Autodesk Inventor part; units mm, degrees
(part 2 of 7)
sketch "Sketch1" plane through (0, 0, 0) normal (0, 0, 1) x (1, 0, 0)
  circle A0 centre (3.25, 6.65) radius 1.2295 projected
  line L0 (0, 0) -> (6.5, 0) projected
  line L1 (6.5, 0) -> (6.5, 9.3) projected
  line L2 (6.5, 9.3) -> (0, 9.3) projected
  line L3 (0, 0) -> (0, 9.3) projected
  circle A1 centre (3.25, 13.15) radius 1.2295 projected
  line L4 (0, 9.3) -> (6.5, 9.3) projected
  line L5 (6.5, 9.3) -> (6.5, 17) projected
  line L6 (0, 17) -> (6.5, 17) projected
  line L7 (0, 9.3) -> (0, 17) projected
  circle A2 centre (-9.75, 13.15) radius 1.2295 projected
  line L8 (-41.3371, 11.3) -> (-13, 11.3) projected
  line L9 (-41.3371, 9.3) -> (-41.3371, 11.3) projected
  line L10 (-41.3371, 9.3) -> (-6.5, 9.3) projected
  line L11 (-6.5, 9.3) -> (-6.5, 17) projected
  line L12 (-13, 17) -> (-6.5, 17) projected
  line L13 (-13, 11.3) -> (-13, 17) projected
  circle A3 centre (-9.75, -51.55) radius 1.2295 projected
  line L14 (-41.3371, -47.7) -> (-6.5, -47.7) projected
  line L15 (-41.3371, -47.7) -> (-41.3371, -49.7) projected
  line L16 (-13, -49.7) -> (-41.3371, -49.7) projected
  line L17 (-13, -49.7) -> (-13, -55.4) projected
  line L18 (-6.5, -55.4) -> (-13, -55.4) projected
  line L19 (-6.5, -47.7) -> (-6.5, -55.4) projected
  circle A4 centre (3.25, -51.55) radius 1.2295 projected
  line L20 (0, -47.7) -> (6.5, -47.7) projected
  line L21 (0, -47.7) -> (0, -55.4) projected
  line L22 (6.5, -55.4) -> (0, -55.4) projected
  line L23 (6.5, -47.7) -> (6.5, -55.4) projected
  circle A5 centre (3.25, -45.05) radius 1.2295 projected
  line L24 (0.5983, -42.4) -> (0, -42.4) projected
  line L25 (0, -42.4) -> (0, -47.7) projected
  line L26 (0, -47.7) -> (6.5, -47.7) projected
  line L27 (6.5, -38.4) -> (6.5, -47.7) projected
  line L28 (0.5983, -38.4) -> (6.5, -38.4) projected
  line L29 (0.5983, -38.4) -> (0.5983, -42.4) projected
  arc A6 (-64.7971, 16.2257) -> (-64.1621, 16.7072) centre (-64.6621, 16.7072) ccw projected
  line L30 (-64.1621, 16.7072) -> (-64.1621, 23.8) projected
  arc A7 (-64.1621, 23.8) -> (-67.1621, 26.8) centre (-67.1621, 23.8) ccw projected
  line L31 (-67.1621, 26.8) -> (-70.1621, 26.8) projected
  line L32 (-70.1621, 26.8) -> (-70.1621, 29.3) projected
  line L33 (-70.1621, 29.3) -> (-59.3371, 29.3) projected
  line L34 (-59.3371, 29.3) -> (-59.3371, 30.8) projected
  line L35 (-59.3371, 30.8) -> (-78.8451, 30.8) projected
  line L36 (-78.8451, 16.3) -> (-78.8451, 30.8) projected
  line L37 (-65.3371, 16.3) -> (-78.8451, 16.3) projected
  arc A8 (-64.7971, 16.2257) -> (-65.3371, 16.3) centre (-65.3371, 14.3) ccw projected
  circle A9 centre (-67.4121, 21.8) radius 1.2295 projected
  circle A10 centre (-74.1621, 21.8) radius 1.2295 projected
  circle A11 centre (-67.4121, -60.2) radius 1.2295 projected
  circle A12 centre (-74.1621, -60.2) radius 1.2295 projected
  arc A13 (-64.1621, -55.1072) -> (-64.7971, -54.6257) centre (-64.6621, -55.1072) ccw projected
  arc A14 (-65.3371, -54.7) -> (-64.7971, -54.6257) centre (-65.3371, -52.7) ccw projected
  line L38 (-65.3371, -54.7) -> (-78.8451, -54.7) projected
  line L39 (-78.8451, -54.7) -> (-78.8451, -69.2) projected
  line L40 (-59.3371, -69.2) -> (-78.8451, -69.2) projected
  line L41 (-59.3371, -67.7) -> (-59.3371, -69.2) projected
  line L42 (-59.3371, -67.7) -> (-70.1621, -67.7) projected
  line L43 (-70.1621, -67.7) -> (-70.1621, -65.2) projected
  line L44 (-70.1621, -65.2) -> (-67.1621, -65.2) projected
  arc A15 (-67.1621, -65.2) -> (-64.1621, -62.2) centre (-67.1621, -62.2) ccw projected
  line L45 (-64.1621, -62.2) -> (-64.1621, -55.1072) projected
  line L46 (-78.5805, 30.8) -> (-78.5805, -69.2) projected
  line L47 (-78.3805, 30.8) -> (-78.3805, -69.2)
  line L48 (-41.3371, 11.3) -> (-41.3371, 30.8)
  line L49 (-41.3371, 30.8) -> (-59.3371, 30.8)
  line L50 (-41.3371, -49.7) -> (-41.3371, -69.2)
  line L51 (-41.3371, -69.2) -> (-59.3371, -69.2)
  line L52 (-6.5, 17) -> (0, 17)
  line L53 (-6.5, -55.4) -> (0, -55.4)
  line L54 (-15.8027, 0.2) -> (-0.5973, 0.2)
  line L55 (-0.5973, 0.2) -> (-0.5973, -38.6)
  line L56 (-0.5973, -38.6) -> (-15.8027, -38.6)
  line L57 (-15.8027, -38.6) -> (-15.8027, 0.2)
  line L58 (-56.7398, 0.2) -> (-41.5344, 0.2)
  line L59 (-41.5344, 0.2) -> (-41.5344, -38.6)
  line L60 (-41.5344, -38.6) -> (-56.7398, -38.6)
  line L61 (-56.7398, -38.6) -> (-56.7398, 0.2)
  line L62 (6.3, 17) -> (6.3, -55.4)
  line L63 (-24.219, -0.425) -> (-24.469, -0.675) construction
  line L64 (-24.469, -0.675) -> (-24.469, -0.725) construction
  line L65 (-24.469, -0.725) -> (-24.569, -0.725) construction
  line L66 (-24.569, -5.125) -> (-24.569, -0.725) construction
  line L67 (-24.469, -5.125) -> (-24.569, -5.125) construction
  line L68 (-24.469, -5.125) -> (-24.469, -5.175) construction
  line L69 (-24.469, -5.175) -> (-24.219, -5.425) construction
  line L70 (-24.219, -5.425) -> (-23.369, -5.425) construction
  line L71 (-23.369, -5.925) -> (-23.369, -5.425) construction
  line L72 (-21.669, -5.925) -> (-23.369, -5.925) construction
  line L73 (-21.669, -5.925) -> (-21.669, 0.075) construction
  line L74 (-21.669, 0.075) -> (-23.369, 0.075) construction
  line L75 (-23.369, 0.075) -> (-23.369, -0.425) construction
  line L76 (-24.219, -0.425) -> (-23.369, -0.425) construction
  line L77 (-24.269, -5.225) -> (-23.169, -5.225) construction
  line L78 (-24.269, -0.625) -> (-24.269, -5.225) construction
  line L79 (-24.269, -0.625) -> (-23.169, -0.625) construction
  line L80 (-23.169, -0.625) -> (-23.169, -0.375) construction
  line L81 (-22.569, -0.375) -> (-23.169, -0.375) construction
  line L82 (-22.569, -0.375) -> (-22.569, -0.625) construction
  line L83 (-22.569, -0.625) -> (-21.969, -0.625) construction
  line L84 (-21.969, -5.225) -> (-21.969, -0.625) construction
  line L85 (-22.569, -5.225) -> (-21.969, -5.225) construction
  line L86 (-22.569, -5.475) -> (-22.569, -5.225) construction
  line L87 (-22.569, -5.475) -> (-23.169, -5.475) construction
  line L88 (-23.169, -5.225) -> (-23.169, -5.475) construction
  line L89 (-30.969, -4.8) -> (-30.719, -4.55) construction
  line L90 (-30.719, -4.55) -> (-30.719, -4.5) construction
  line L91 (-30.719, -4.5) -> (-30.619, -4.5) construction
  line L92 (-30.619, -0.1) -> (-30.619, -4.5) construction
  line L93 (-30.719, -0.1) -> (-30.619, -0.1) construction
  line L94 (-30.719, -0.1) -> (-30.719, -0.05) construction
  line L95 (-30.719, -0.05) -> (-30.969, 0.2) construction
  line L96 (-30.969, 0.2) -> (-31.819, 0.2) construction
  line L97 (-31.819, 0.7) -> (-31.819, 0.2) construction
  line L98 (-33.519, 0.7) -> (-31.819, 0.7) construction
  line L99 (-33.519, 0.7) -> (-33.519, -5.3) construction
  line L100 (-33.519, -5.3) -> (-31.819, -5.3) construction
  line L101 (-31.819, -5.3) -> (-31.819, -4.8) construction
  line L102 (-30.969, -4.8) -> (-31.819, -4.8) construction
  line L103 (-30.919, 0) -> (-32.019, 0) construction
  line L104 (-30.919, -4.6) -> (-30.919, 0) construction
  line L105 (-30.919, -4.6) -> (-32.019, -4.6) construction
  line L106 (-32.019, -4.6) -> (-32.019, -4.85) construction
  line L107 (-32.619, -4.85) -> (-32.019, -4.85) construction
  line L108 (-32.619, -4.85) -> (-32.619, -4.6) construction
  line L109 (-32.619, -4.6) -> (-33.219, -4.6) construction
  line L110 (-33.219, 0) -> (-33.219, -4.6) construction
  line L111 (-32.619, 0) -> (-33.219, 0) construction
  line L112 (-32.619, 0.25) -> (-32.619, 0) construction
  line L113 (-32.619, 0.25) -> (-32.019, 0.25) construction
  line L114 (-32.019, 0) -> (-32.019, 0.25) construction
  line L115 (-30.6923, 2.9785) -> (-30.6409, 3.0299) construction
  line L116 (-28.244, -45.725) -> (-28.244, -46.975) construction
  line L117 (-27.894, -45.725) -> (-28.244, -45.725) construction
  line L118 (-27.894, -40.225) -> (-27.894, -45.725) construction
  line L119 (-27.894, -40.225) -> (-28.244, -40.225) construction
  line L120 (-28.244, -40.225) -> (-28.244, -38.975) construction
  line L121 (-28.7932, -38.975) -> (-28.244, -38.975) construction
  line L122 (-28.7932, -38.975) -> (-30.4948, -38.975) construction
  line L123 (-30.4948, -38.975) -> (-31.044, -38.975) construction
  line L124 (-31.044, -40.225) -> (-31.044, -38.975) construction
  line L125 (-31.394, -40.225) -> (-31.044, -40.225) construction
  line L126 (-31.394, -40.225) -> (-31.394, -45.725) construction
  line L127 (-31.394, -45.725) -> (-31.044, -45.725) construction
  line L128 (-31.044, -45.725) -> (-31.044, -46.975) construction
  line L129 (-30.4948, -46.975) -> (-31.044, -46.975) construction
  line L130 (-28.7932, -46.975) -> (-30.4948, -46.975) construction
  line L131 (-28.7932, -46.975) -> (-28.244, -46.975) construction
  line L132 (-30.7278, -45.075) -> (-30.7278, -40.875) construction
  line L133 (-30.7278, -40.875) -> (-28.5602, -40.875) construction
  line L134 (-28.5602, -45.075) -> (-28.5602, -40.875) construction
  line L135 (-30.7278, -45.075) -> (-28.5602, -45.075) construction
  line L136 (-26.369, -32.525) -> (-26.619, -32.775) construction
  line L137 (-26.619, -32.775) -> (-26.619, -32.825) construction
  line L138 (-26.619, -32.825) -> (-26.719, -32.825) construction
  line L139 (-26.719, -37.225) -> (-26.719, -32.825) construction
  line L140 (-26.619, -37.225) -> (-26.719, -37.225) construction
  line L141 (-26.619, -37.225) -> (-26.619, -37.275) construction
  line L142 (-26.619, -37.275) -> (-26.369, -37.525) construction
  line L143 (-26.369, -37.525) -> (-25.519, -37.525) construction
  line L144 (-25.519, -38.025) -> (-25.519, -37.525) construction
  line L145 (-23.819, -38.025) -> (-25.519, -38.025) construction
  line L146 (-23.819, -38.025) -> (-23.819, -32.025) construction
  line L147 (-23.819, -32.025) -> (-25.519, -32.025) construction
  line L148 (-25.519, -32.025) -> (-25.519, -32.525) construction
  line L149 (-26.369, -32.525) -> (-25.519, -32.525) construction
  line L150 (-26.419, -37.325) -> (-25.319, -37.325) construction
  line L151 (-26.419, -32.725) -> (-26.419, -37.325) construction
  line L152 (-26.419, -32.725) -> (-25.319, -32.725) construction
  line L153 (-25.319, -32.725) -> (-25.319, -32.475) construction
  line L154 (-24.719, -32.475) -> (-25.319, -32.475) construction
  line L155 (-24.719, -32.475) -> (-24.719, -32.725) construction
  line L156 (-24.719, -32.725) -> (-24.119, -32.725) construction
  line L157 (-24.119, -37.325) -> (-24.119, -32.725) construction
  line L158 (-24.719, -37.325) -> (-24.119, -37.325) construction
  line L159 (-24.719, -37.575) -> (-24.719, -37.325) construction
  line L160 (-24.719, -37.575) -> (-25.319, -37.575) construction
  line L161 (-25.319, -37.325) -> (-25.319, -37.575) construction
  line L162 (-39.469, 6.6787) -> (-39.469, 5.7213) construction
  line L163 (-38.769, 5.7213) -> (-39.469, 5.7213) construction
  line L164 (-38.769, 6.6787) -> (-38.769, 5.7213) construction
  line L165 (-38.769, 6.6787) -> (-39.469, 6.6787) construction
  line L166 (-41.644, 6.7037) -> (-41.644, 5.7463) construction
  line L167 (-40.944, 5.7463) -> (-41.644, 5.7463) construction
  line L168 (-40.944, 6.7037) -> (-40.944, 5.7463) construction
  line L169 (-40.944, 6.7037) -> (-41.644, 6.7037) construction
  line L170 (-43.869, 6.6659) -> (-43.869, 5.7085) construction
  line L171 (-43.169, 5.7085) -> (-43.869, 5.7085) construction
  line L172 (-43.169, 6.6659) -> (-43.169, 5.7085) construction
  line L173 (-43.169, 6.6659) -> (-43.869, 6.6659) construction
  circle A16 centre (-17.024, 4.925) radius 0.4 construction
  line L174 (-48.969, 4.8) -> (-48.969, 8.75) construction
  line L175 (-45.019, 4.8) -> (-48.969, 4.8) construction
  line L176 (-45.019, 8.75) -> (-45.019, 4.8) construction
  line L177 (-48.969, 8.75) -> (-45.019, 8.75) construction
  line L178 (-17.974, -6.7) -> (-30.974, -6.7) construction
  line L179 (-30.974, -6.7) -> (-30.974, -31.3) construction
  line L180 (-30.974, -31.3) -> (-17.974, -31.3) construction
  line L181 (-17.974, -31.3) -> (-17.974, -6.7) construction
  line L182 (-19.0216, -29.9049) -> (-19.0216, -8.0951) construction
  line L183 (-29.9264, -29.9049) -> (-19.0216, -29.9049) construction
  line L184 (-29.9264, -8.0951) -> (-29.9264, -29.9049) construction
  line L185 (-19.0216, -8.0951) -> (-29.9264, -8.0951) construction
  line L186 (-12.8905, 1.2342) -> (-8.9405, 1.2342) construction
  line L187 (-8.9405, 1.2342) -> (-8.9405, 5.1842) construction
  line L188 (-8.9405, 5.1842) -> (-12.8905, 5.1842) construction
  line L189 (-12.8905, 5.1842) -> (-12.8905, 1.2342) construction
  line L190 (-20.8623, -46.6822) -> (-16.9123, -46.6822) construction
  line L191 (-16.9123, -46.6822) -> (-16.9123, -42.7322) construction
  line L192 (-16.9123, -42.7322) -> (-20.8623, -42.7322) construction
  line L193 (-20.8623, -42.7322) -> (-20.8623, -46.6822) construction
  line L194 (-8.9405, 5.1842) -> (-12.8905, 1.2342) construction
  line L195 (-12.8905, 5.1842) -> (-8.9405, 1.2342) construction
  line L196 (-13.5155, 5.8092) -> (-8.3155, 5.8092)
  line L197 (-8.3155, 5.8092) -> (-8.3155, 0.6092)
  line L198 (-8.3155, 0.6092) -> (-13.5155, 0.6092)
  line L199 (-13.5155, 0.6092) -> (-13.5155, 5.8092)
  line L200 (-13.5155, 5.8092) -> (-8.3155, 0.6092) construction
  line L201 (-8.3155, 5.8092) -> (-13.5155, 0.6092) construction
  line L202 (-45.019, 8.75) -> (-48.969, 4.8) construction
  line L203 (-48.969, 8.75) -> (-45.019, 4.8) construction
  line L204 (-20.9331, -46.753) -> (-16.9123, -42.7322) construction
  line L205 (-20.8623, -42.7322) -> (-16.9123, -46.6822) construction
  line L206 (-49.994, 9.775) -> (-43.994, 9.775)
  line L207 (-43.994, 9.775) -> (-43.994, 3.775)
  line L208 (-43.994, 3.775) -> (-49.994, 3.775)
  line L209 (-49.994, 3.775) -> (-49.994, 9.775)
  line L210 (-49.994, 9.775) -> (-43.994, 3.775) construction
  line L211 (-43.994, 9.775) -> (-49.994, 3.775) construction
  line L212 (-21.4873, -42.1072) -> (-16.2873, -42.1072)
  line L213 (-16.2873, -42.1072) -> (-16.2873, -47.3072)
  line L214 (-16.2873, -47.3072) -> (-21.4873, -47.3072)
  line L215 (-21.4873, -47.3072) -> (-21.4873, -42.1072)
  line L216 (-21.4873, -42.1072) -> (-16.2873, -47.3072) construction
  line L217 (-16.2873, -42.1072) -> (-21.4873, -47.3072) construction
  circle A17 centre (-27.2755, 4.5435) radius 1.595 construction
  circle A18 centre (-27.2755, 4.5435) radius 4.5
  line L218 (-20.869, 1.575) -> (-25.369, 1.575)
  line L219 (-25.369, 1.575) -> (-25.369, -6.5)
  line L220 (-25.369, -6.5) -> (-20.869, -6.5)
  line L221 (-20.869, -6.5) -> (-20.869, 1.575)
  line L222 (-34.319, 2.2) -> (-29.819, 2.2)
  line L223 (-29.819, 2.2) -> (-29.819, -6.5)
  line L224 (-29.819, -6.5) -> (-34.319, -6.5)
  line L225 (-34.319, -6.5) -> (-34.319, 2.2)
  line L226 (-27.519, -39.525) -> (-23.019, -39.525)
  line L227 (-23.019, -39.525) -> (-23.019, -31.5)
  line L228 (-23.019, -31.5) -> (-27.519, -31.5)
  line L229 (-27.519, -31.5) -> (-27.519, -39.525)
  line L230 (-43.994, 7.6787) -> (-37.769, 7.6787)
  line L231 (-37.769, 7.6787) -> (-37.769, 4.7213)
  line L232 (-43.994, 3.775) -> (-43.994, 7.6787)
  circle A19 centre (-17.024, 4.925) radius 1
  line L233 (-27.144, -38.225) -> (-32.144, -38.225)
  line L234 (-32.144, -38.225) -> (-32.144, -47.7)
  line L235 (-32.144, -47.7) -> (-27.144, -47.7)
  line L236 (-27.144, -47.7) -> (-27.144, -38.225)
  line L237 (-17.8027, -6.5) -> (-34.8027, -6.5)
  line L238 (-34.8027, -6.5) -> (-34.8027, -31.5)
  line L239 (-34.8027, -31.5) -> (-17.8027, -31.5)
  line L240 (-17.8027, -31.5) -> (-17.8027, -6.5)
  line L241 (-37.769, 4.7213) -> (-43.994, 4.7213)
  line L242 (-14.0915, 0) -> (-2.3085, 0)
  line L243 (-2.3085, -38.4) -> (-14.0915, -38.4)
  line L244 (-43.2456, -38.4) -> (-55.0286, -38.4)
  line L245 (-55.0286, 0) -> (-43.2456, 0)
  line L246 (-41.7344, -5.25) -> (-41.7344, -33.15)
  line L247 (-56.5398, -33.15) -> (-56.5398, -5.25)
  line L248 (-0.7973, -5.25) -> (-0.7973, -33.15)
  line L249 (-15.6027, -33.15) -> (-15.6027, -5.25)
  line L250 (-14.0915, 0) -> (-2.3085, 0)
  line L251 (-2.3085, -38.4) -> (-14.0915, -38.4)
  line L252 (-2.1085, 0.2) -> (-2.1085, -4.25)
  line L253 (-2.1085, -4.25) -> (-0.5973, -4.25)
  line L254 (-2.1085, -38.6) -> (-2.1085, -34.15)
  line L255 (-2.1085, -34.15) -> (-0.5973, -34.15)
  line L256 (-14.2915, -38.6) -> (-14.2915, -34.15)
  line L257 (-14.2915, -34.15) -> (-15.8027, -34.15)
  line L258 (-43.0456, 0.2) -> (-43.0456, -4.25)
  line L259 (-43.0456, -4.25) -> (-41.5344, -4.25)
  line L260 (-55.2286, 0.2) -> (-55.2286, -4.25)
  line L261 (-55.2286, -4.25) -> (-56.7398, -4.25)
  line L262 (-56.7398, -34.15) -> (-55.2286, -34.15)
  line L263 (-55.2286, -34.15) -> (-55.2286, -38.6)
  line L264 (-41.5344, -34.15) -> (-43.0456, -34.15)
  line L265 (-43.0456, -34.15) -> (-43.0456, -38.6)
  line L266 (-14.2915, 0.2) -> (-14.2915, -4.25)
  line L267 (-14.2915, -4.25) -> (-15.8027, -4.25)
  line L268 (-13, 17) -> (-13, 30.8)
  line L269 (-13, 30.8) -> (6.3, 30.8)
  line L270 (6.3, 30.8) -> (6.3, 17)
  line L271 (-13, -55.4) -> (-13, -69.2)
  line L272 (-13, -69.2) -> (6.3, -69.2)
  line L273 (6.3, -69.2) -> (6.3, -55.4)
  point P0 (-10.9155, 3.2092)
  point P1 (-46.994, 6.775)
  point P2 (-18.8873, -44.7072)
  point P3 (-25.369, 0.4673)
  point P4 (-29.819, 0.8313)
  point P5 (-27.519, -38.225)
  point P6 (-31.1171, 2.2)
  point P7 (-23.8935, 1.575)
  point P8 (-27.144, -39.525)
  dimension "d0" = 0.2
  dimension "d9" = 0.2
  dimension "d12" = 5.2
  dimension "d13" = 5.2
  dimension "d14" = 6
  dimension "d15" = 6
  dimension "d16" = 5.2
  dimension "d17" = 5.2
  dimension "d18" = 9
  dimension "d20" = 1
  dimension "d21" = 1
  dimension "d23" = 0.125
  dimension "d24" = 1.5
  dimension "d25" = 1.2
  dimension "d26" = 0.8
  dimension "d27" = 0.8
  dimension "d28" = 1.5
  dimension "d29" = 0.8
  dimension "d30" = 0.8
  dimension "d31" = 0.575
  dimension "d32" = 1.5
  dimension "d33" = 0.8
  dimension "d34" = 0.8
  dimension "d35" = 0.525
  dimension "d36" = 4.5
  dimension "d37" = 8.7
  dimension "d38" = 2
  dimension "d41" = 0.75
  dimension "d42" = 0.75
  dimension "d43" = 0.725
  dimension "d44" = 0.75
  dimension "d45" = 1.5951
  dimension "d46" = 1.5951
  dimension "d47" = 25
  dimension "d48" = 17
  dimension "d49" = 2
  dimension "d51" = 1
  dimension "d54" = 0.2
  dimension "d55" = 0.2
  dimension "d56" = 0.2
  dimension "d57" = 0.2
  dimension "d58" = 0.2
  dimension "d59" = 0.2
  dimension "d60" = 0.2
  dimension "d61" = 0.2
  dimension "d64" = 0.2
  dimension "d65" = 0.2
  dimension "d66" = 0.2
  dimension "d67" = 0.2
  dimension "d68" = 0.2
  dimension "d69" = 0.2
  dimension "d70" = 0.2
  dimension "d71" = 0.2
  dimension "d72" = 1
  dimension "d73" = 1
  dimension "d74" = 1
  dimension "d75" = 1
  dimension "d76" = 1
  dimension "d77" = 1
  dimension "d78" = 1
  dimension "d79" = 1
  constraints: 192 end point, 37 perpendicular, 27 point on line, 22 parallel, 20 horizontal, 9 midpoint, 7 vertical, 2 centre point, 2 coincident, 2 collinear, 16 other
  measures "d0" distance between parallel lines of L47 L46
  measures "d9" distance between parallel lines of L62 L1
  measures "d12" distance of L197.end L198.end
  measures "d13" distance of L196.end L197.end
  measures "d14" distance of L207.end L208.end
  measures "d15" distance of L206.end L207.end
  measures "d16" distance of L213.end L214.end
  measures "d17" distance of L212.end L213.end
  measures "d18" diameter of A18
  measures "d20" distance from line of L230 L164.start
  measures "d21" distance from line of L231 L164.start
  measures "d23" distance from line of L232 L170.end
  measures "d24" distance from line of L222 L98.start
  measures "d25" distance from line of L224 L99.end
  measures "d26" distance from line of L225 L98.start
  measures "d27" distance from line of L223 L92.start
  measures "d28" distance from line of L218 L73.end
  measures "d29" distance from line of L219 L65.end
  measures "d30" distance from line of L221 L72.start
  measures "d31" distance from line of L220 L72.start
  measures "d32" distance from line of L226 L145.start
  measures "d33" distance from line of L227 L145.start
  measures "d34" distance from line of L229 L138.end
  measures "d35" distance from line of L228 L147.end
  measures "d36" distance between parallel lines of L225 L223
  measures "d37" distance between parallel lines of L222 L224
  measures "d38" diameter of A19
  measures "d41" distance from line of L233 L120.end
  measures "d42" distance from line of L236 L118.start
  measures "d43" distance from line of L14 L116.end
  measures "d44" distance from line of L234 L125.start
  measures "d45" distance from line of L237 L182.end
  measures "d46" distance from line of L239 L182.start
  measures "d47" distance of L239.end L237.start
  measures "d48" distance between parallel lines of L240 L238
  measures "d49" distance between parallel lines of L240 L57
  measures "d51" distance from line of L241 L163.start
  measures "d54" distance between parallel lines of L54 L242
  measures "d55" distance between parallel lines of L56 L243
  measures "d56" distance between parallel lines of L60 L244
  measures "d57" distance between parallel lines of L58 L245
  measures "d58" distance between parallel lines of L55 L248
  measures "d59" distance between parallel lines of L57 L249
  measures "d60" distance between parallel lines of L59 L246
  measures "d61" distance between parallel lines of L247 L61
  measures "d64" distance from line of L245.end L258
  measures "d65" distance from line of L260 L245.start
  measures "d66" distance from line of L263 L244.end
  measures "d67" distance from line of L265 L244.start
  measures "d68" distance from line of L256 L243.end
  measures "d69" distance from line of L243.start L254
  measures "d70" distance from line of L242.start L266
  measures "d71" distance from line of L252 L242.end
  measures "d72" distance from line of L248.start L253
  measures "d73" distance from line of L267 L249.end
  measures "d74" distance from line of L249.start L257
  measures "d75" distance from line of L248.end L255
  measures "d76" distance from line of L246.end L264
  measures "d77" distance from line of L247.start L262
  measures "d78" distance from line of L247.end L261
  measures "d79" distance from line of L259 L246.start
extrude "Extrusion1" add sketch "Sketch1" along normal blind 2 contours A0 | L3 L2 L62 L0 | L0 L62 L28 L29 L24 L25 L21 L53 L19 L14 L236 L226 L227 L239 L240 L237 L221 L218 A18 L222 L225 L238 L229 L233 L234 L15 L50 L51 L41 L42 L43 L44 A15 L45 A13 A14 L38 L47 L37 A8 A6 L30 A7 L31 L32 L33 L34 L49 L48 L9 L10 L11 L52 L7 L3 | L7 L6 L62 L2 | L62 L20 L25 L24 L29 L28 | L62 L22 L21 L20 | L11 L10 L9 L8 L13 L12 | L18 L17 L16 L15 L14 L19 | L34 L33 L32 L31 A7 L30 A6 A8 L37 L47 L35 | L40 L47 L38 A14 A13 L45 A15 L44 L43 L42 L41 | A1 | A2 | A3 | A4 | A5 | A9 | A10 | A11 | A12
fillet "Fillet1" radius 0.5 30 edges at (-23.8935, 1.575, 1) (-20.869, 1.575, 1) (-20.869, -6.5, 1) (-31.1171, 2.2, 1) (-34.319, 2.2, 1) (-34.8027, -6.5, 1) (-27.519, -31.5, 1) (-23.019, -31.5, 1) (-23.019, -39.525, 1) (-27.144, -39.525, 1) (-27.519, -38.225, 1) (-43.994, 7.6787, 1) (-37.769, 7.6787, 1) (-37.769, 4.7213, 1) (-43.994, 4.7213, 1) (-43.994, 3.775, 1) (-43.994, 9.775, 1) (-49.994, 9.775, 1) (-49.994, 3.775, 1) (-34.319, -6.5, 1) (-41.3371, 30.8, 1) (-41.3371, -69.2, 1) (-56.7398, 0.2, 1) (-41.5344, 0.2, 1) (-41.5344, -38.6, 1) (-56.7398, -38.6, 1) (-15.8027, -38.6, 1) (-0.5973, -38.6, 1) (-0.5973, 0.2, 1) (-15.8027, 0.2, 1)
sketch "Sketch2" plane through (0, 0, 2) normal (0, 0, 1) x (1, 0, 0)
  circle A0 centre (3.25, 13.15) radius 1.2295 projected
  line L0 (0, 9.3) -> (6.5, 9.3) projected
  line L1 (6.5, 9.3) -> (6.5, 17) projected
  line L2 (0, 17) -> (6.5, 17) projected
  line L3 (0, 9.3) -> (0, 17) projected
  circle A1 centre (3.25, 6.65) radius 1.2295 projected
  line L4 (0, 0) -> (6.5, 0) projected
  line L5 (6.5, 0) -> (6.5, 9.3) projected
  line L6 (6.5, 9.3) -> (0, 9.3) projected
  line L7 (0, 0) -> (0, 9.3) projected
  circle A2 centre (-9.75, 13.15) radius 1.2295 projected
  line L8 (-41.3371, 11.3) -> (-13, 11.3) projected
  line L9 (-41.3371, 9.3) -> (-41.3371, 11.3) projected
  line L10 (-41.3371, 9.3) -> (-6.5, 9.3) projected
  line L11 (-6.5, 9.3) -> (-6.5, 17) projected
  line L12 (-13, 17) -> (-6.5, 17) projected
  line L13 (-13, 11.3) -> (-13, 17) projected
  circle A3 centre (3.25, -45.05) radius 1.2295 projected
  line L14 (0.5983, -42.4) -> (0, -42.4) projected
  line L15 (0, -42.4) -> (0, -47.7) projected
  line L16 (0, -47.7) -> (6.5, -47.7) projected
  line L17 (6.5, -38.4) -> (6.5, -47.7) projected
  line L18 (0.5983, -38.4) -> (6.5, -38.4) projected
  line L19 (0.5983, -38.4) -> (0.5983, -42.4) projected
  circle A4 centre (3.25, -51.55) radius 1.2295 projected
  line L20 (0, -47.7) -> (6.5, -47.7) projected
  line L21 (0, -47.7) -> (0, -55.4) projected
  line L22 (6.5, -55.4) -> (0, -55.4) projected
  line L23 (6.5, -47.7) -> (6.5, -55.4) projected
  circle A5 centre (-9.75, -51.55) radius 1.2295 projected
  line L24 (-41.3371, -47.7) -> (-6.5, -47.7) projected
  line L25 (-41.3371, -47.7) -> (-41.3371, -49.7) projected
  line L26 (-13, -49.7) -> (-41.3371, -49.7) projected
  line L27 (-13, -49.7) -> (-13, -55.4) projected
  line L28 (-6.5, -55.4) -> (-13, -55.4) projected
  line L29 (-6.5, -47.7) -> (-6.5, -55.4) projected
  circle A6 centre (-67.4121, -60.2) radius 1.2295 projected
  circle A7 centre (-74.1621, -60.2) radius 1.2295 projected
  arc A8 (-64.1621, -55.1072) -> (-64.7971, -54.6257) centre (-64.6621, -55.1072) ccw projected
  arc A9 (-65.3371, -54.7) -> (-64.7971, -54.6257) centre (-65.3371, -52.7) ccw projected
  line L30 (-65.3371, -54.7) -> (-78.8451, -54.7) projected
  line L31 (-78.8451, -54.7) -> (-78.8451, -69.2) projected
  line L32 (-59.3371, -69.2) -> (-78.8451, -69.2) projected
  line L33 (-59.3371, -67.7) -> (-59.3371, -69.2) projected
  line L34 (-59.3371, -67.7) -> (-70.1621, -67.7) projected
  line L35 (-70.1621, -67.7) -> (-70.1621, -65.2) projected
  line L36 (-70.1621, -65.2) -> (-67.1621, -65.2) projected
  arc A10 (-67.1621, -65.2) -> (-64.1621, -62.2) centre (-67.1621, -62.2) ccw projected
  line L37 (-64.1621, -62.2) -> (-64.1621, -55.1072) projected
  arc A11 (-64.7971, 16.2257) -> (-64.1621, 16.7072) centre (-64.6621, 16.7072) ccw projected
  line L38 (-64.1621, 16.7072) -> (-64.1621, 23.8) projected
  arc A12 (-64.1621, 23.8) -> (-67.1621, 26.8) centre (-67.1621, 23.8) ccw projected
  line L39 (-67.1621, 26.8) -> (-70.1621, 26.8) projected
  line L40 (-70.1621, 26.8) -> (-70.1621, 29.3) projected
  line L41 (-70.1621, 29.3) -> (-59.3371, 29.3) projected
  line L42 (-59.3371, 29.3) -> (-59.3371, 30.8) projected
  line L43 (-59.3371, 30.8) -> (-78.8451, 30.8) projected
  line L44 (-78.8451, 16.3) -> (-78.8451, 30.8) projected
  line L45 (-65.3371, 16.3) -> (-78.8451, 16.3) projected
  arc A13 (-64.7971, 16.2257) -> (-65.3371, 16.3) centre (-65.3371, 14.3) ccw projected
  circle A14 centre (-67.4121, 21.8) radius 1.2295 projected
  circle A15 centre (-74.1621, 21.8) radius 1.2295 projected
hole "Hole1" at (-74.1621, 21.8, 2) at (-67.4121, 21.8, 2) at (-74.1621, -60.2, 2) at (-67.4121, -60.2, 2) at (-9.75, 13.15, 2) at (3.25, 13.15, 2) at (3.25, 6.65, 2) at (3.25, -45.05, 2) at (3.25, -51.55, 2) at (-9.75, -51.55, 2) direction (0, 0, -1) diameter 3 depth 7.6 clearance for "Countersunk Flat Head Screw ISO 2009/7046" size "M3" standard "ISO"
sketch "Sketch3" plane through (0, 0, 2) normal (0, 0, 1) x (1, 0, 0)
  circle A0 centre (-9.75, -51.55) radius 1.5 projected
  circle A1 centre (3.25, -51.55) radius 1.5 projected
  circle A2 centre (3.25, -45.05) radius 1.5 projected
  circle A3 centre (3.25, 6.65) radius 1.5 projected
  circle A4 centre (3.25, 13.15) radius 1.5 projected
  circle A5 centre (-9.75, 13.15) radius 1.5 projected
  circle A6 centre (-67.4121, -60.2) radius 1.5 projected
  circle A7 centre (-74.1621, -60.2) radius 1.5 projected
  circle A8 centre (-67.4121, 21.8) radius 1.5 projected
  circle A9 centre (-74.1621, 21.8) radius 1.5 projected
  arc A10 (-34.5609, -6.5715) -> (-34.319, -6.1433) centre (-34.819, -6.1433) ccw projected
  line L0 (-34.319, -6.1433) -> (-34.319, 1.7) projected
  arc A11 (-33.819, 2.2) -> (-34.319, 1.7) centre (-33.819, 1.7) ccw projected
  line L1 (-33.819, 2.2) -> (-31.9232, 2.2) projected
  arc A12 (-31.9232, 2.2) -> (-31.4585, 2.8843) centre (-31.9232, 2.7) ccw projected
  arc A13 (-23.3621, 2.3219) -> (-31.4585, 2.8843) centre (-27.2755, 4.5435) ccw projected
  arc A14 (-23.3621, 2.3219) -> (-22.9273, 1.575) centre (-22.9273, 2.075) ccw projected
  line L2 (-22.9273, 1.575) -> (-21.369, 1.575) projected
  arc A15 (-20.869, 1.075) -> (-21.369, 1.575) centre (-21.369, 1.075) ccw projected
  line L3 (-20.869, 1.075) -> (-20.869, -6) projected
  arc A16 (-20.869, -6) -> (-20.369, -6.5) centre (-20.369, -6) ccw projected
  line L4 (-20.369, -6.5) -> (-17.8027, -6.5) projected
  line L5 (-17.8027, -6.5) -> (-17.8027, -31.5) projected
  line L6 (-17.8027, -31.5) -> (-22.519, -31.5) projected
  arc A17 (-22.519, -31.5) -> (-23.019, -32) centre (-22.519, -32) ccw projected
  line L7 (-23.019, -32) -> (-23.019, -39.025) projected
  arc A18 (-23.519, -39.525) -> (-23.019, -39.025) centre (-23.519, -39.025) ccw projected
  line L8 (-23.519, -39.525) -> (-26.644, -39.525) projected
  arc A19 (-26.644, -39.525) -> (-27.144, -40.025) centre (-26.644, -40.025) ccw projected
  line L9 (-27.144, -40.025) -> (-27.144, -47.7) projected
  line L10 (-27.144, -47.7) -> (-32.144, -47.7) projected
  line L11 (-32.144, -47.7) -> (-32.144, -38.225) projected
  line L12 (-32.144, -38.225) -> (-28.019, -38.225) projected
  arc A20 (-28.019, -38.225) -> (-27.519, -37.725) centre (-28.019, -37.725) ccw projected
  line L13 (-27.519, -37.725) -> (-27.519, -32) projected
  arc A21 (-27.519, -32) -> (-28.019, -31.5) centre (-28.019, -32) ccw projected
  line L14 (-28.019, -31.5) -> (-34.8027, -31.5) projected
  line L15 (-34.8027, -31.5) -> (-34.8027, -6.9997) projected
  arc A22 (-34.5609, -6.5715) -> (-34.8027, -6.9997) centre (-34.3027, -6.9997) ccw projected
  arc A23 (-41.8371, -69.2) -> (-41.3371, -68.7) centre (-41.8371, -68.7) ccw projected
  line L16 (-41.3371, -68.7) -> (-41.3371, -49.7) projected
  line L17 (-41.3371, -49.7) -> (-13, -49.7) projected
  line L18 (-13, -49.7) -> (-13, -55.4) projected
  line L19 (-13, -55.4) -> (6.3, -55.4) projected
  line L20 (6.3, -55.4) -> (6.3, 17) projected
  line L21 (6.3, 17) -> (-13, 17) projected
  line L22 (-13, 17) -> (-13, 11.3) projected
  line L23 (-13, 11.3) -> (-41.3371, 11.3) projected
  line L24 (-41.3371, 11.3) -> (-41.3371, 30.3) projected
  arc A24 (-41.3371, 30.3) -> (-41.8371, 30.8) centre (-41.8371, 30.3) ccw projected
  line L25 (-41.8371, 30.8) -> (-78.3805, 30.8) projected
  line L26 (-78.3805, 30.8) -> (-78.3805, -69.2) projected
  line L27 (-78.3805, -69.2) -> (-41.8371, -69.2) projected
  line L28 (-56.7398, -38.1) -> (-56.7398, -0.3) projected
  line L29 (-56.2398, 0.2) -> (-42.0344, 0.2) projected
  line L30 (-41.5344, -0.3) -> (-41.5344, -38.1) projected
  line L31 (-42.0344, -38.6) -> (-56.2398, -38.6) projected
  line L32 (-15.3027, 0.2) -> (-1.0973, 0.2) projected
  line L33 (-0.5973, -0.3) -> (-0.5973, -38.1) projected
  line L34 (-1.0973, -38.6) -> (-15.3027, -38.6) projected
  line L35 (-15.8027, -38.1) -> (-15.8027, -0.3) projected
  arc A25 (-44.4926, 3.775) -> (-43.9933, 4.2482) centre (-44.4926, 4.275) ccw projected
  line L36 (-44.4926, 3.775) -> (-49.494, 3.775) projected
  arc A26 (-49.994, 4.275) -> (-49.494, 3.775) centre (-49.494, 4.275) ccw projected
  line L37 (-49.994, 4.275) -> (-49.994, 9.275) projected
  arc A27 (-49.494, 9.775) -> (-49.994, 9.275) centre (-49.494, 9.275) ccw projected
  line L38 (-49.494, 9.775) -> (-44.494, 9.775) projected
  arc A28 (-43.994, 9.275) -> (-44.494, 9.775) centre (-44.494, 9.275) ccw projected
  line L39 (-43.994, 9.275) -> (-43.994, 8.1787) projected
  arc A29 (-43.994, 8.1787) -> (-43.494, 7.6787) centre (-43.494, 8.1787) ccw projected
  line L40 (-43.494, 7.6787) -> (-38.269, 7.6787) projected
  arc A30 (-37.769, 7.1787) -> (-38.269, 7.6787) centre (-38.269, 7.1787) ccw projected
  line L41 (-37.769, 7.1787) -> (-37.769, 5.2213) projected
  arc A31 (-38.269, 4.7213) -> (-37.769, 5.2213) centre (-38.269, 5.2213) ccw projected
  line L42 (-38.269, 4.7213) -> (-43.494, 4.7213) projected
  arc A32 (-43.494, 4.7213) -> (-43.9933, 4.2482) centre (-43.494, 4.2213) ccw projected
  line L43 (-13.5155, 5.8092) -> (-8.3155, 5.8092) projected
  line L44 (-8.3155, 5.8092) -> (-8.3155, 0.6092) projected
  line L45 (-8.3155, 0.6092) -> (-13.5155, 0.6092) projected
  line L46 (-13.5155, 0.6092) -> (-13.5155, 5.8092) projected
  line L47 (-21.4873, -42.1072) -> (-16.2873, -42.1072) projected
  line L48 (-16.2873, -42.1072) -> (-16.2873, -47.3072) projected
  line L49 (-16.2873, -47.3072) -> (-21.4873, -47.3072) projected
  line L50 (-21.4873, -47.3072) -> (-21.4873, -42.1072) projected
  circle A33 centre (-17.024, 4.925) radius 1 projected
  circle A34 centre (-67.4121, 21.8) radius 3.25
  circle A35 centre (-74.1621, 21.8) radius 3.25
  circle A36 centre (-67.4121, -60.2) radius 3.25
  circle A37 centre (-74.1621, -60.2) radius 3.25
  circle A38 centre (-9.75, -51.55) radius 3.25
  circle A39 centre (3.25, -51.55) radius 3.25
  circle A40 centre (3.25, -45.05) radius 3.25
  circle A41 centre (3.25, 6.65) radius 3.25
  circle A42 centre (3.25, 13.15) radius 3.25
  circle A43 centre (-9.75, 13.15) radius 3.25
  line L51 (-61.7398, 30.8) -> (-61.7398, -69.2) construction
  line L52 (-61.7398, -69.2) -> (-71.5197, -69.2) construction
  line L53 (-71.5197, -69.2) -> (-71.5197, 30.8) construction
  line L54 (-71.5197, 30.8) -> (-61.7398, 30.8) construction
  line L55 (-55.7398, 30.8) -> (-55.7398, 0.2) construction
  line L56 (-55.7398, 0.2) -> (-61.7398, 0.2) construction
  line L57 (-61.7398, 0.2) -> (-61.7398, 30.8) construction
  line L58 (-61.7398, 30.8) -> (-55.7398, 30.8) construction
  line L59 (-72.8805, -1.2) -> (-72.8805, -69.2) construction
  line L60 (-72.8805, -69.2) -> (-78.3805, -69.2) construction
  line L61 (-78.3805, -69.2) -> (-78.3805, -1.2) construction
  line L62 (-78.3805, -1.2) -> (-72.8805, -1.2) construction
  line L63 (6.3, 17) -> (6.3, -55.4) construction
  line L64 (6.3, -55.4) -> (0.4027, -55.4) construction
  line L65 (0.4027, -55.4) -> (0.4027, 17) construction
  line L66 (0.4027, 17) -> (6.3, 17) construction
  line L67 (6.3, -55.4) -> (6.3, 17) projected
  line L68 (6.3, 17) -> (-13, 17) projected
  line L69 (-13, -55.4) -> (6.3, -55.4) projected
  line L70 (-34.8027, 11.3) -> (-34.8027, -49.7) construction
  line L71 (-34.8027, -49.7) -> (-41.5344, -49.7) construction
  line L72 (-41.5344, -49.7) -> (-41.5344, 11.3) construction
  line L73 (-41.5344, 11.3) -> (-34.8027, 11.3) construction
  line L74 (-13, 11.3) -> (-41.3371, 11.3) projected
  line L75 (20.4964, 29.5628) -> (19.2617, 25.9997)
  line L76 (19.2617, 25.9997) -> (18.8736, 24.8576)
  line L77 (18.8736, 24.8576) -> (19.0632, 24.7149)
  line L78 (19.0632, 24.7149) -> (19.5439, 24.6945)
  line L79 (19.5439, 24.6945) -> (19.9904, 24.7711)
  line L80 (19.9904, 24.7711) -> (20.3641, 25.0428)
  line L81 (20.3641, 25.0428) -> (21.1314, 26.4231)
  line L82 (-51.3968, 25.8193) -> (-52.0652, 26.0877)
  arc A44 (-52.0652, 26.0877) -> (-52.0252, 25.6948) centre (-51.9558, 25.9004) ccw
  line L83 (-78.3805, -64.2) -> (-41.3371, -64.2) construction
  line L84 (-41.3371, -64.2) -> (-41.3371, -69.2) construction
  line L85 (-41.3371, -69.2) -> (-78.3805, -69.2) construction
  line L86 (-78.3805, -69.2) -> (-78.3805, -64.2) construction
  arc A45 (-0.5973, -0.3) -> (-1.0973, 0.2) centre (-1.0973, -0.3) ccw projected
  arc A46 (-1.0973, -38.6) -> (-0.5973, -38.1) centre (-1.0973, -38.1) ccw projected
  arc A47 (-15.8027, -38.1) -> (-15.3027, -38.6) centre (-15.3027, -38.1) ccw projected
  arc A48 (-15.3027, 0.2) -> (-15.8027, -0.3) centre (-15.3027, -0.3) ccw projected
  arc A49 (-41.5344, -0.3) -> (-42.0344, 0.2) centre (-42.0344, -0.3) ccw projected
  arc A50 (-42.0344, -38.6) -> (-41.5344, -38.1) centre (-42.0344, -38.1) ccw projected
  arc A51 (-56.7398, -38.1) -> (-56.2398, -38.6) centre (-56.2398, -38.1) ccw projected
  arc A52 (-56.2398, 0.2) -> (-56.7398, -0.3) centre (-56.2398, -0.3) ccw projected
  line L87 (-43.0973, 21.0657) -> (-43.3928, 21.709)
  line L88 (-43.3928, 21.709) -> (-43.7204, 22.2677)
  line L89 (-43.7204, 22.2677) -> (-44.0527, 22.5468)
  line L90 (-44.0527, 22.5468) -> (-44.3747, 22.736)
  line L91 (-44.3747, 22.736) -> (-45.2196, 23.1839)
  line L92 (-45.2196, 23.1839) -> (-46.252, 23.7057)
  line L93 (-46.252, 23.7057) -> (-46.6961, 23.8893)
  line L94 (-46.6961, 23.8893) -> (-47.0155, 23.9884)
  line L95 (-47.0155, 23.9884) -> (-47.1564, 24.0454)
  line L96 (-47.1564, 24.0454) -> (-47.7937, 24.3584)
  line L97 (-47.7937, 24.3584) -> (-48.6002, 24.6932)
  line L98 (-48.6002, 24.6932) -> (-49.9175, 25.2277)
  line L99 (-49.9175, 25.2277) -> (-51.3968, 25.8193)
  line L100 (-52.0252, 25.6948) -> (-51.5813, 25.5448)
  line L101 (-51.5813, 25.5448) -> (-51.358, 25.4849)
  line L102 (-51.358, 25.4849) -> (-50.9261, 25.3244)
  line L103 (-50.9261, 25.3244) -> (-49.7216, 24.8106)
  line L104 (-49.7216, 24.8106) -> (-48.7354, 24.4045)
  line L105 (-48.7354, 24.4045) -> (-47.862, 24.0482)
  line L106 (-47.862, 24.0482) -> (-46.8407, 23.6137)
  line L107 (-46.8407, 23.6137) -> (-45.852, 23.1688)
  line L108 (-45.852, 23.1688) -> (-44.8057, 22.5966)
  line L109 (-44.8057, 22.5966) -> (-44.4801, 22.4154)
  line L110 (-44.4801, 22.4154) -> (-44.2916, 22.3405)
  line L111 (-44.2916, 22.3405) -> (-44.1568, 22.2781)
  line L112 (-44.1568, 22.2781) -> (-43.9901, 22.0986)
  line L113 (-43.9901, 22.0986) -> (-43.7987, 21.8117)
  line L114 (-43.7987, 21.8117) -> (-43.5897, 21.4275)
  line L115 (-43.5897, 21.4275) -> (-43.4509, 21.1367)
  line L116 (-43.4509, 21.1367) -> (-43.3713, 20.9143)
  line L117 (-43.3713, 20.9143) -> (-43.3367, 20.7012)
  line L118 (-43.3367, 20.7012) -> (-43.3327, 20.4387)
  line L119 (-43.3327, 20.4387) -> (-43.3767, 19.7818)
  line L120 (-43.3767, 19.7818) -> (-43.4569, 19.3738)
  line L121 (-43.4569, 19.3738) -> (-43.5854, 18.9863)
  line L122 (-43.5854, 18.9863) -> (-43.7936, 18.5005)
  line L123 (-43.7936, 18.5005) -> (-44.1286, 17.9107)
  line L124 (-44.1286, 17.9107) -> (-44.5098, 17.3449)
  line L125 (-44.5098, 17.3449) -> (-44.8566, 16.9311)
  line L126 (-44.8566, 16.9311) -> (-45.2403, 16.5876)
  line L127 (-45.2403, 16.5876) -> (-45.6158, 16.3115)
  line L128 (-45.6158, 16.3115) -> (-45.9672, 16.1121)
  line L129 (-45.9672, 16.1121) -> (-46.2786, 15.9985)
  line L130 (-46.2786, 15.9985) -> (-46.7506, 15.9386)
  line L131 (-46.7506, 15.9386) -> (-47.4502, 15.8903)
  line L132 (-47.4502, 15.8903) -> (-48.3041, 15.8443)
  line L133 (-48.3041, 15.8443) -> (-48.4868, 16.0355)
  line L134 (-48.4868, 16.0355) -> (-48.6386, 16.2701)
  line L135 (-48.6386, 16.2701) -> (-48.8063, 16.633)
  line L136 (-48.8063, 16.633) -> (-48.9698, 17.0753)
  line L137 (-48.9698, 17.0753) -> (-49.1087, 17.5479)
  line L138 (-49.1087, 17.5479) -> (-49.1671, 17.9451)
  line L139 (-49.1671, 17.9451) -> (-49.1406, 18.3947)
  line L140 (-49.1406, 18.3947) -> (-49.0427, 19.0452)
  line L141 (-49.0427, 19.0452) -> (-48.9463, 19.3465)
  line L142 (-48.9463, 19.3465) -> (-48.8248, 19.734)
  line L143 (-48.8248, 19.734) -> (-48.7427, 19.9228)
  line L144 (-48.7427, 19.9228) -> (-48.6019, 20.108)
  line L145 (-48.6019, 20.108) -> (-48.4307, 20.2573)
  line L146 (-48.4307, 20.2573) -> (-48.2579, 20.3385)
  line L147 (-48.2579, 20.3385) -> (-48.1306, 20.4095)
  line L148 (-48.1306, 20.4095) -> (-48.0878, 20.5284)
  line L149 (-48.0878, 20.5284) -> (-48.0943, 20.6035)
  line L150 (-48.0943, 20.6035) -> (-48.1208, 20.6423)
  line L151 (-48.1208, 20.6423) -> (-48.2708, 20.6349)
  line L152 (-48.2708, 20.6349) -> (-48.4766, 20.5502)
  line L153 (-48.4766, 20.5502) -> (-48.7091, 20.418)
  line L154 (-48.7091, 20.418) -> (-48.8521, 20.3267)
  line L155 (-48.8521, 20.3267) -> (-48.946, 20.2928)
  line L156 (-48.946, 20.2928) -> (-49.029, 20.3131)
  line L157 (-49.029, 20.3131) -> (-49.1396, 20.3844)
  line L158 (-49.1396, 20.3844) -> (-49.3537, 20.4935)
  line L159 (-49.3537, 20.4935) -> (-49.7014, 20.623)
  line L160 (-49.7014, 20.623) -> (-50.4854, 20.8414)
  line L161 (-50.4854, 20.8414) -> (-50.8379, 20.9204)
  line L162 (-50.8379, 20.9204) -> (-51.2901, 20.9848)
  line L163 (-51.2901, 20.9848) -> (-52.2132, 21.067)
  line L164 (-52.2132, 21.067) -> (-52.9747, 21.183)
  line L165 (-52.9747, 21.183) -> (-53.1401, 21.2025)
  line L166 (-53.1401, 21.2025) -> (-53.2667, 21.1656)
  line L167 (-53.2667, 21.1656) -> (-53.3233, 21.0901)
  line L168 (-53.3233, 21.0901) -> (-53.2788, 20.9937)
  line L169 (-53.2788, 20.9937) -> (-53.1471, 20.912)
  line L170 (-53.1471, 20.912) -> (-52.9213, 20.8512)
  line L171 (-52.9213, 20.8512) -> (-52.0028, 20.7487)
  line L172 (-52.0028, 20.7487) -> (-51.1482, 20.6427)
  line L173 (-51.1482, 20.6427) -> (-50.3026, 20.472)
  line L174 (-50.3026, 20.472) -> (-49.6145, 20.2728)
  line L175 (-49.6145, 20.2728) -> (-49.376, 20.1738)
  line L176 (-49.376, 20.1738) -> (-49.2326, 20.0814)
  line L177 (-49.2326, 20.0814) -> (-49.1448, 19.9803)
  line L178 (-49.1448, 19.9803) -> (-49.1099, 19.8939)
  line L179 (-49.1099, 19.8939) -> (-49.1227, 19.7813)
  line L180 (-49.1227, 19.7813) -> (-49.1781, 19.6014)
  line L181 (-49.1781, 19.6014) -> (-49.3806, 18.8791)
  line L182 (-49.3806, 18.8791) -> (-49.4737, 18.2364)
  line L183 (-49.4737, 18.2364) -> (-49.4566, 17.6925)
  line L184 (-49.4566, 17.6925) -> (-49.4065, 17.4636)
  line L185 (-49.4065, 17.4636) -> (-49.3285, 17.2666)
  line L186 (-49.3285, 17.2666) -> (-49.2588, 17.0688)
  line L187 (-49.2588, 17.0688) -> (-49.2499, 16.9453)
  line L188 (-49.2499, 16.9453) -> (-49.1485, 16.652)
  line L189 (-49.1485, 16.652) -> (-48.8538, 16.0229)
  line L190 (-48.8538, 16.0229) -> (-48.6845, 15.7938)
  line L191 (-48.6845, 15.7938) -> (-48.5307, 15.6547)
  line L192 (-48.5307, 15.6547) -> (-48.2288, 15.6059)
  line L193 (-48.2288, 15.6059) -> (-47.6755, 15.5878)
  line L194 (-47.6755, 15.5878) -> (-47.0347, 15.6011)
  line L195 (-47.0347, 15.6011) -> (-46.4705, 15.6464)
  line L196 (-46.4705, 15.6464) -> (-46.0987, 15.7274)
  line L197 (-46.0987, 15.7274) -> (-45.742, 15.8693)
  line L198 (-45.742, 15.8693) -> (-45.3942, 16.0747)
  line L199 (-45.3942, 16.0747) -> (-45.0495, 16.3463)
  line L200 (-45.0495, 16.3463) -> (-44.6358, 16.7208)
  line L201 (-44.6358, 16.7208) -> (-44.3421, 17.0243)
  line L202 (-44.3421, 17.0243) -> (-44.1239, 17.307)
  line L203 (-44.1239, 17.307) -> (-43.9366, 17.6189)
  line L204 (-43.9366, 17.6189) -> (-43.6525, 18.1046)
  line L205 (-43.6525, 18.1046) -> (-43.523, 18.3069)
  line L206 (-43.523, 18.3069) -> (-43.3617, 18.6996)
  line L207 (-43.3617, 18.6996) -> (-43.2066, 19.1823)
  line L208 (-43.2066, 19.1823) -> (-43.0959, 19.6546)
  line L209 (-43.0959, 19.6546) -> (-43.0398, 20.0564)
  line L210 (-43.0398, 20.0564) -> (-43.0222, 20.4472)
  line L211 (-43.0222, 20.4472) -> (-43.0417, 20.7944)
  line L212 (-43.0417, 20.7944) -> (-43.0973, 21.0657)
  line L213 (-45.7764, 18.0496) -> (-45.8933, 18.1577)
  line L214 (-45.8933, 18.1577) -> (-45.9298, 18.1594)
  line L215 (-45.9298, 18.1594) -> (-45.9525, 18.1279)
  line L216 (-45.9525, 18.1279) -> (-45.9994, 18.0796)
  line L217 (-45.9994, 18.0796) -> (-46.0515, 18.079)
  line L218 (-46.0515, 18.079) -> (-46.1283, 18.0616)
  line L219 (-46.1283, 18.0616) -> (-46.2213, 17.9597)
  line L220 (-46.2213, 17.9597) -> (-46.2942, 17.8189)
  line L221 (-46.2942, 17.8189) -> (-46.2717, 17.7714)
  line L222 (-46.2717, 17.7714) -> (-46.2081, 17.7197)
  line L223 (-46.2081, 17.7197) -> (-46.0985, 17.6494)
  line L224 (-46.0985, 17.6494) -> (-46.0012, 17.6307)
  line L225 (-46.0012, 17.6307) -> (-45.8998, 17.6649)
  line L226 (-45.8998, 17.6649) -> (-45.7776, 17.7533)
  line L227 (-45.7776, 17.7533) -> (-45.6289, 17.8868)
  line L228 (-45.6289, 17.8868) -> (-45.7764, 18.0496)
  line L229 (-50.2693, 16.6848) -> (-50.9232, 17.2377)
  line L230 (-50.9232, 17.2377) -> (-51.3215, 17.568)
  line L231 (-51.3215, 17.568) -> (-51.7783, 18.0076)
  line L232 (-51.7783, 18.0076) -> (-53.2491, 19.6107)
  line L233 (-53.2491, 19.6107) -> (-53.5909, 19.9446)
  line L234 (-53.5909, 19.9446) -> (-53.7148, 20.0243)
  line L235 (-53.7148, 20.0243) -> (-53.8118, 20.0504)
  line L236 (-53.8118, 20.0504) -> (-53.9256, 20.0367)
  line L237 (-53.9256, 20.0367) -> (-53.8756, 19.9801)
  line L238 (-53.8756, 19.9801) -> (-53.8193, 19.9314)
  line L239 (-53.8193, 19.9314) -> (-53.8265, 19.9093)
  line L240 (-53.8265, 19.9093) -> (-53.7889, 19.8131)
  line L241 (-53.7889, 19.8131) -> (-53.6091, 19.5839)
  line L242 (-53.6091, 19.5839) -> (-53.3854, 19.2823)
  line L243 (-53.3854, 19.2823) -> (-53.3518, 19.1652)
  line L244 (-53.3518, 19.1652) -> (-53.3572, 19.0396)
  line L245 (-53.3572, 19.0396) -> (-53.7947, 15.5136)
  line L246 (-53.7947, 15.5136) -> (-53.8063, 15.279)
  line L247 (-53.8063, 15.279) -> (-53.7749, 15.1819)
  line L248 (-53.7749, 15.1819) -> (-53.3651, 15.3143)
  line L249 (-53.3651, 15.3143) -> (-52.9492, 15.4449)
  line L250 (-52.9492, 15.4449) -> (-52.454, 15.5646)
  line L251 (-52.454, 15.5646) -> (-51.8054, 15.7225)
  line L252 (-51.8054, 15.7225) -> (-51.1005, 15.9331)
  line L253 (-51.1005, 15.9331) -> (-50.5, 16.1442)
  line L254 (-50.5, 16.1442) -> (-50.165, 16.3033)
  line L255 (-50.165, 16.3033) -> (-49.9951, 16.4297)
  line L256 (-49.9951, 16.4297) -> (-50.2693, 16.6848)
  line L257 (-51.0336, 16.1022) -> (-52.5089, 15.7104)
  line L258 (-52.5089, 15.7104) -> (-53.2554, 15.5426)
  line L259 (-53.2554, 15.5426) -> (-53.5973, 15.4916)
  line L260 (-53.5973, 15.4916) -> (-53.5616, 16.0265)
  line L261 (-53.5616, 16.0265) -> (-53.4283, 17.1675)
  line L262 (-53.4283, 17.1675) -> (-53.2683, 18.3468)
  line L263 (-53.2683, 18.3468) -> (-53.1528, 18.9965)
  line L264 (-53.1528, 18.9965) -> (-52.9595, 18.8264)
  line L265 (-52.9595, 18.8264) -> (-52.5133, 18.3589)
  line L266 (-52.5133, 18.3589) -> (-51.707, 17.5381)
  line L267 (-51.707, 17.5381) -> (-50.763, 16.722)
  line L268 (-50.763, 16.722) -> (-50.5151, 16.5069)
  line L269 (-50.5151, 16.5069) -> (-50.4627, 16.4313)
  line L270 (-50.4627, 16.4313) -> (-50.4619, 16.368)
  line L271 (-50.4619, 16.368) -> (-50.5157, 16.3102)
  line L272 (-50.5157, 16.3102) -> (-50.627, 16.2512)
  line L273 (-50.627, 16.2512) -> (-51.0336, 16.1022)
  line L274 (-51.7978, 17.3259) -> (-51.9942, 17.6027)
  line L275 (-51.9942, 17.6027) -> (-52.1487, 17.7789)
  line L276 (-52.1487, 17.7789) -> (-52.2663, 17.8528)
  line L277 (-52.2663, 17.8528) -> (-52.2947, 17.8492)
  line L278 (-52.2947, 17.8492) -> (-52.3029, 17.8218)
  line L279 (-52.3029, 17.8218) -> (-52.2592, 17.7059)
  line L280 (-52.2592, 17.7059) -> (-52.1356, 17.5248)
  line L281 (-52.1356, 17.5248) -> (-51.9251, 17.2559)
  line L282 (-51.9251, 17.2559) -> (-52.0668, 17.0871)
  line L283 (-52.0668, 17.0871) -> (-52.2016, 16.9183)
  line L284 (-52.2016, 16.9183) -> (-52.2433, 17.0666)
  line L285 (-52.2433, 17.0666) -> (-52.2942, 17.1568)
  line L286 (-52.2942, 17.1568) -> (-52.3724, 17.2153)
  line L287 (-52.3724, 17.2153) -> (-52.4441, 17.2262)
  line L288 (-52.4441, 17.2262) -> (-52.4757, 17.1734)
  line L289 (-52.4757, 17.1734) -> (-52.4135, 16.995)
  line L290 (-52.4135, 16.995) -> (-52.2703, 16.7263)
  line L291 (-52.2703, 16.7263) -> (-52.1124, 16.4814)
  line L292 (-52.1124, 16.4814) -> (-52.0062, 16.3742)
  line L293 (-52.0062, 16.3742) -> (-51.9399, 16.3837)
  line L294 (-51.9399, 16.3837) -> (-51.9205, 16.4197)
  line L295 (-51.9205, 16.4197) -> (-52.0194, 16.6142)
  line L296 (-52.0194, 16.6142) -> (-52.0729, 16.7053)
  line L297 (-52.0729, 16.7053) -> (-52.0849, 16.7705)
  line L298 (-52.0849, 16.7705) -> (-51.9758, 16.9103)
  line L299 (-51.9758, 16.9103) -> (-51.8494, 16.9918)
  line L300 (-51.8494, 16.9918) -> (-51.8138, 16.9861)
  line L301 (-51.8138, 16.9861) -> (-51.7922, 16.9519)
  line L302 (-51.7922, 16.9519) -> (-51.7413, 16.8956)
  line L303 (-51.7413, 16.8956) -> (-51.6638, 16.8676)
  line L304 (-51.6638, 16.8676) -> (-51.5941, 16.8727)
  line L305 (-51.5941, 16.8727) -> (-51.5666, 16.9157)
  line L306 (-51.5666, 16.9157) -> (-51.7978, 17.3259)
  line L307 (-52.4853, 16.5525) -> (-52.6361, 16.5567)
  line L308 (-52.6361, 16.5567) -> (-52.782, 16.455)
  line L309 (-52.782, 16.455) -> (-52.8723, 16.3355)
  line L310 (-52.8723, 16.3355) -> (-52.8771, 16.2639)
  line L311 (-52.8771, 16.2639) -> (-52.8116, 16.2596)
  line L312 (-52.8116, 16.2596) -> (-52.6907, 16.3417)
  line L313 (-52.6907, 16.3417) -> (-52.5799, 16.4236)
  line L314 (-52.5799, 16.4236) -> (-52.5158, 16.4283)
  line L315 (-52.5158, 16.4283) -> (-52.5022, 16.3578)
  line L316 (-52.5022, 16.3578) -> (-52.5431, 16.2141)
  line L317 (-52.5431, 16.2141) -> (-52.5744, 16.0714)
  line L318 (-52.5744, 16.0714) -> (-52.5519, 15.9919)
  line L319 (-52.5519, 15.9919) -> (-52.4934, 15.9917)
  line L320 (-52.4934, 15.9917) -> (-52.4166, 16.0866)
  line L321 (-52.4166, 16.0866) -> (-52.3535, 16.2474)
  line L322 (-52.3535, 16.2474) -> (-52.3448, 16.3853)
  line L323 (-52.3448, 16.3853) -> (-52.3892, 16.4903)
  line L324 (-52.3892, 16.4903) -> (-52.4853, 16.5525)
  line L325 (-42.2022, -46.9293) -> (-42.5931, -47.4343)
  line L326 (-42.5931, -47.4343) -> (-42.9399, -47.8571)
  line L327 (-42.9399, -47.8571) -> (-43.2647, -48.2227)
  line L328 (-43.2647, -48.2227) -> (-43.5891, -48.5562)
  line L329 (-43.5891, -48.5562) -> (-44.132, -49.0542)
  line L330 (-44.132, -49.0542) -> (-44.3978, -49.2679)
  line L331 (-44.3978, -49.2679) -> (-44.6664, -49.4625)
  line L332 (-44.6664, -49.4625) -> (-44.9424, -49.6412)
  line L333 (-44.9424, -49.6412) -> (-45.2307, -49.8072)
  line L334 (-45.2307, -49.8072) -> (-45.8636, -50.1145)
  line L335 (-45.8636, -50.1145) -> (-46.298, -50.3164)
  line L336 (-46.298, -50.3164) -> (-46.2075, -50.4417)
  line L337 (-46.2075, -50.4417) -> (-45.9627, -50.7126)
  line L338 (-45.9627, -50.7126) -> (-45.6311, -51.0769)
  line L339 (-45.6311, -51.0769) -> (-45.3526, -51.4261)
  line L340 (-45.3526, -51.4261) -> (-45.1221, -51.7681)
  line L341 (-45.1221, -51.7681) -> (-44.934, -52.1109)
  line L342 (-44.934, -52.1109) -> (-44.7821, -52.4663)
  line L343 (-44.7821, -52.4663) -> (-44.6759, -52.8224)
  line L344 (-44.6759, -52.8224) -> (-44.6082, -53.2114)
  line L345 (-44.6082, -53.2114) -> (-44.5721, -53.6654)
  line L346 (-44.5721, -53.6654) -> (-44.5454, -54.1912)
  line L347 (-44.5454, -54.1912) -> (-44.9035, -54.1683)
  line L348 (-44.9035, -54.1683) -> (-45.2583, -54.1231)
  line L349 (-45.2583, -54.1231) -> (-45.6189, -54.035)
  line L350 (-45.6189, -54.035) -> (-45.9751, -53.9069)
  line L351 (-45.9751, -53.9069) -> (-46.317, -53.7416)
  line L352 (-46.317, -53.7416) -> (-46.3421, -53.7579)
  line L353 (-46.3421, -53.7579) -> (-46.3818, -53.8152)
  line L354 (-46.3818, -53.8152) -> (-46.4809, -54.0021)
  line L355 (-46.4809, -54.0021) -> (-46.5656, -54.1997)
  line L356 (-46.5656, -54.1997) -> (-46.5875, -54.3055)
  line L357 (-46.5875, -54.3055) -> (-44.0615, -56.1838)
  line L358 (-44.0615, -56.1838) -> (-43.4018, -56.6872)
  line L359 (-43.4018, -56.6872) -> (-42.7047, -57.242)
  line L360 (-42.7047, -57.242) -> (-42.1525, -57.7011)
  line L361 (-42.1525, -57.7011) -> (-41.9879, -57.8488)
  line L362 (-41.9879, -57.8488) -> (-41.9279, -57.9174)
  line L363 (-41.9279, -57.9174) -> (-41.9604, -57.9743)
  line L364 (-41.9604, -57.9743) -> (-42.0703, -58.0555)
  line L365 (-42.0703, -58.0555) -> (-42.5985, -58.3365)
  line L366 (-42.5985, -58.3365) -> (-43.4224, -58.7192)
  line L367 (-43.4224, -58.7192) -> (-43.8037, -58.8735)
  line L368 (-43.8037, -58.8735) -> (-44.1749, -59.0065)
  line L369 (-44.1749, -59.0065) -> (-44.5435, -59.1208)
  line L370 (-44.5435, -59.1208) -> (-44.9173, -59.2189)
  line L371 (-44.9173, -59.2189) -> (-45.7112, -59.3766)
  line L372 (-45.7112, -59.3766) -> (-46.0236, -59.4146)